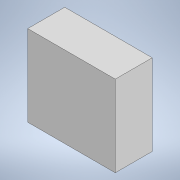
# Autodesk Inventor part: AndymarkBattery
Saved by Autodesk Inventor 2022 (Build 260153000, 153)
## iProperties
Created: 2022-01-10
Part Number: AndymarkBattery
Material: Generic
Document SubType Name: Modeling
Designer: merky
Density: 1 g/cm^3
Appearance: Default
Author: merky
Autodesk Inventor part; units mm, degrees
ref_plane "YZ Plane" through (0, 0, 0) normal (1, 0, 0) x (0, 1, 0)
ref_plane "XZ Plane" through (0, 0, 0) normal (0, 1, 0) x (-1, 0, 0)
ref_plane "XY Plane" through (0, 0, 0) normal (0, 0, 1) x (1, 0, 0)
sketch "Sketch1" plane through (0, 0, 0) normal (0, 1, 0) x (-1, 0, 0)
  line L0 (0, 0) -> (180.34, 0)
  line L1 (180.34, 0) -> (180.34, -76.2)
  line L2 (180.34, -76.2) -> (0, -76.2)
  line L3 (0, -76.2) -> (0, 0)
  dimension "d0" = 180.34
  dimension "d1" = 76.2
  constraints: 8 end point, 2 parallel, 1 horizontal, 1 perpendicular
  measures "d0" distance of L1.end L2.end
  measures "d1" distance of L0.end L1.end
extrude "Extrusion1" add sketch "Sketch1" along normal blind 167.132
sketch "Sketch2" plane through (0, 0, 0) normal (0, -1, 0) x (1, 0, 0)
  line L0 (-180.34, -76.2) -> (-180.34, 0) projected
  line L1 (-193.04, 0) -> (-193.04, -76.2)
  line L2 (-193.04, -76.2) -> (-180.34, -76.2)
  line L3 (-180.34, -76.2) -> (-180.34, 0)
  line L4 (0, -76.2) -> (-180.34, -76.2) projected
  line L5 (0, -76.2) -> (12.7, -76.2)
  line L6 (12.7, -76.2) -> (12.7, 0)
  line L7 (0, 0) -> (0, -76.2)
  line L8 (0, 0) -> (-180.34, 0)
  line L9 (-193.04, 0) -> (-193.04, 12.7)
  line L10 (-193.04, 12.7) -> (12.7, 12.7)
  line L11 (12.7, 12.7) -> (12.7, 0)
  dimension "d4" = 12.7
  dimension "d5" = 12.7
  dimension "d6" = 12.7
  constraints: 20 end point, 4 parallel, 2 horizontal, 2 perpendicular, 1 point on line
  measures "d4" distance of L2.end L1.end
  measures "d5" distance of L7.start L6.end
  measures "d6" distance of L9.start L9.end
body "Solid1"
